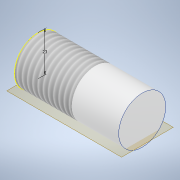
# Autodesk Inventor part: Cilindro Inicial con Corte
Saved by Autodesk Inventor 2021 (Build 250183000, 183)
## iProperties
Created: 2021-01-01
Part Number: Cilindro Inicial con Corte
Material: Aluminum 6061
Document SubType Name: Modeling
Designer: dieku
Density: 2.7 g/cm^3
Appearance: Aluminum - Flat
Author: dieku
Autodesk Inventor part; units mm, degrees
ref_plane "YZ Plane" through (0, 0, 0) normal (1, 0, 0) x (0, 1, 0)
ref_plane "XY Plane" through (0, 0, 0) normal (0, 0, 1) x (1, 0, 0)
sketch "Sketch1" plane through (0, 0, 0) normal (0, 0, 1) x (1, 0, 0)
  line L0 (0, 0) -> (0, 13.5)
  line L1 (0, 13.5) -> (60, 13.5)
  line L2 (60, 13.5) -> (60, 0)
  line L3 (60, 0) -> (0, 0)
  line L4 (0, 0) -> (64.8862, 0) construction
  dimension "d0" = 13.5
  dimension "d1" = 60
  constraints: 10 end point, 2 horizontal, 2 vertical, 1 perpendicular
  measures "d0" distance of L0.start L0.end
  measures "d1" distance of L0.end L1.end
revolve "Revolution3" add sketch "Sketch1" angle 360 about axis through (0, 0, 0) along (1, 0, 0)
ref_plane "Work Plane3" through (0, -9.5, 0) normal (0, 1, 0) x (-1, 0, 0)
sketch "Sketch5" plane through (0, -9.5, 0) normal (0, 1, 0) x (-1, 0, 0)
  line L0 (0, 0) -> (-33, 0) construction
  line L1 (-33, 0) -> (-36.5, 0) construction
  line L2 (-36.5, 0) -> (-56.5, 0) construction
  line L3 (-46.5, 0) -> (-40.5, 0)
  line L4 (-40.5, 0) -> (-52.5, 0)
  arc A0 (-40.5, -4) -> (-40.5, 4) centre (-40.5, 0) ccw
  arc A1 (-52.5, 4) -> (-52.5, -4) centre (-52.5, 0) ccw
  line L5 (-40.5, -4) -> (-52.5, -4)
  line L6 (-40.5, 4) -> (-52.5, 4)
  dimension "d39" = 33
  dimension "d40" = 3.5
  dimension "d41" = 20
  dimension "d42" = 6
  dimension "d43" = 12
  dimension "d44" = 8
  dimension "d45" = 8
  constraints: 14 end point, 4 point on circle, 3 point on line, 2 centre point, 2 coincident, 2 horizontal, 1 midpoint, 1 parallel, 1 tangent
  measures "d39" distance of L0.start L0.end
  measures "d40" distance of L0.end L1.end
  measures "d41" distance of L1.end L2.end
  measures "d42" distance of L3.start L3.end
  measures "d43" distance of L3.end L4.end
  measures "d44" diameter of A0
  measures "d45" diameter of A1
sketch "Sketch6" plane through (0, 0, 0) normal (-1, 0, 0) x (0, 0, 1)
  circle A0 centre (0, 0) radius 13.5 projected
  line L0 (0, 13.5) -> (0, -9.5)
  line L1 (0, -9.5) -> (9.5917, -9.5)
  line L2 (0, -9.5) -> (-9.5917, -9.5)
  dimension "d46" = 23
  constraints: 6 end point, 3 point on circle, 1 perpendicular, 1 point on line, 1 vertical
  measures "d46" distance of L0.start L0.end
extrude "Extrusion1" cut sketch "Sketch5" against normal blind 4
thread "Thread1" size "M27x3" class "6g" standard "ANSI Metric M Profile" length 33
sketch "Sketch7" plane through (52.5, -9.5, 4) normal (0, 0, -1) x (-1, 0, 0)
  point P0 (52.5, 9.5)
body "Solid3"
